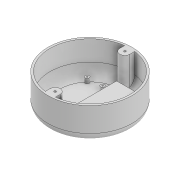
# Autodesk Inventor part: OrTak
Saved by Autodesk Inventor 2022 (Build 260153000, 153)
## iProperties
Created: 2023-02-07
Part Number: OrTak
Material: Generic
Document SubType Name: Modeling
Designer: MVeszpremi
Density: 1 g/cm^3
Appearance: Default
Author: MVeszpremi
Autodesk Inventor part; units mm, degrees
ref_plane "YZ Plane" through (0, 0, 0) normal (1, 0, 0) x (0, 1, 0)
ref_plane "XZ Plane" through (0, 0, 0) normal (0, 1, 0) x (-1, 0, 0)
ref_plane "XY Plane" through (0, 0, 0) normal (0, 0, 1) x (1, 0, 0)
sketch "Sketch1" plane through (0, 0, 0) normal (0, 1, 0) x (-1, 0, 0)
  circle A0 centre (0, 0) radius 62.5
  dimension "d0" = 125
  constraints: 1 centre point, 1 coincident
  measures "d0" diameter of A0
extrude "Extrusion1" add sketch "Sketch1" along normal blind 3
sketch "Sketch2" plane through (0, 3, 0) normal (0, 1, 0) x (1, 0, 0)
  line L0 (-33.1736, -29) -> (-10.1736, -29)
  line L1 (-10.1736, -29) -> (-10.1736, 29)
  line L2 (-10.1736, 29) -> (-33.1736, 29)
  line L3 (-33.1736, 29) -> (-33.1736, -29)
  line L4 (-33.1736, -29) -> (-10.1736, 29) construction
  line L5 (-10.1736, -29) -> (-33.1736, 29) construction
  circle A0 centre (-33.1736, -29) radius 3
  circle A1 centre (-33.1736, 29) radius 3
  circle A2 centre (-10.1736, 29) radius 3
  circle A3 centre (-10.1736, -29) radius 3
  circle A4 centre (-33.1736, -29) radius 0.95
  circle A5 centre (-33.1736, 29) radius 0.95
  circle A6 centre (-10.1736, 29) radius 0.95
  circle A7 centre (-10.1736, -29) radius 0.95
  point P0 (0, 0)
  point P1 (-21.6736, 0)
  dimension "d4" = 58
  dimension "d5" = 23
  dimension "d6" = 6
  dimension "d7" = 6
  dimension "d8" = 6
  dimension "d9" = 6
  dimension "d10" = 1.9
  dimension "d11" = 1.9
  dimension "d12" = 1.9
  dimension "d13" = 1.9
  constraints: 12 end point, 8 centre point, 8 coincident, 2 midpoint, 2 parallel, 1 horizontal, 1 perpendicular
  measures "d4" distance of L2.end L0.start
  measures "d5" distance of L1.end L2.end
  measures "d6" diameter of A0
  measures "d7" diameter of A1
  measures "d8" diameter of A2
  measures "d9" diameter of A3
  measures "d10" diameter of A4
  measures "d11" diameter of A7
  measures "d12" diameter of A6
  measures "d13" diameter of A5
extrude "Extrusion2" add sketch "Sketch2" along normal blind 7 contours A4 L3 A0 L0 | L0 A0 L3 A4 | A3 L1 A7 L0 | L0 A7 L1 A3 | A1 L2 A5 L3 | L3 A5 L2 A1 | A2 L2 A6 L1 | L1 A6 L2 A2
sketch "Sketch3" plane through (0, 3, 0) normal (0, 1, 0) x (1, 0, 0)
  line L0 (12.1501, -27.5) -> (39.6501, -27.5)
  line L1 (39.6501, -27.5) -> (39.6501, 27.5)
  line L2 (39.6501, 27.5) -> (12.1501, 27.5)
  line L3 (12.1501, 27.5) -> (12.1501, -27.5)
  line L4 (12.1501, -27.5) -> (39.6501, 27.5) construction
  line L5 (39.6501, -27.5) -> (12.1501, 27.5) construction
  line L6 (42.6501, -30.5) -> (9.1501, -30.5)
  line L7 (9.1501, -30.5) -> (9.1501, 30.5)
  line L8 (9.1501, 30.5) -> (42.6501, 30.5)
  line L9 (42.6501, 30.5) -> (42.6501, -30.5)
  line L10 (42.6501, -30.5) -> (9.1501, 30.5) construction
  line L11 (9.1501, -30.5) -> (42.6501, 30.5) construction
  circle A0 centre (25.9001, -27.5) radius 10.75
  circle A1 centre (25.9001, -27.5) radius 13.75
  point P0 (0, 0)
  point P1 (25.9001, 0)
  point P2 (15.1501, -27.5)
  point P3 (36.6501, -27.5)
  point P4 (12.4813, -30.5)
  point P5 (39.3188, -30.5)
  dimension "d16" = 55
  dimension "d17" = 27.5
  dimension "d18" = 3
  dimension "d19" = 3
  dimension "d20" = 3
  constraints: 24 end point, 5 midpoint, 4 parallel, 2 horizontal, 2 perpendicular, 1 centre point, 1 coincident, 3 other
  measures "d16" distance of L2.end L0.start
  measures "d17" distance of L1.end L2.end
  measures "d18" distance between parallel lines of L3 L7
  measures "d19" distance between parallel lines of L8 L2
extrude "Extrusion3" cut sketch "Sketch3" against normal blind 7 contours A0 L0 A1 | A0 L6 L0 | L0 A0 | A1 L3 L2 L1 | A0 L6
extrude "Extrusion4" add sketch "Sketch3" along normal blind 19 contours L0 A1 L6 A0 | L1 L2 L3 A1 L6 L7 L8 L9 | A0 L6 A1 L0 | L6 A1 A0
sketch "Sketch4" plane through (0, 22, 0) normal (0, 1, 0) x (1, 0, 0)
  line L0 (39.3188, -30.5) -> (42.6501, -30.5) projected
  line L1 (42.6501, -30.5) -> (42.6501, 30.5) projected
  line L2 (42.6501, 30.5) -> (9.1501, 30.5) projected
  line L3 (9.1501, 30.5) -> (9.1501, -30.5) projected
  line L4 (9.1501, -30.5) -> (12.4813, -30.5) projected
  arc A0 (12.4813, -30.5) -> (39.3188, -30.5) centre (25.9001, -27.5) ccw projected
  arc A1 (15.1501, -27.5) -> (36.6501, -27.5) centre (25.9001, -27.5) ccw projected
  line L5 (15.1501, -27.5) -> (12.1501, -27.5) projected
  line L6 (12.1501, -27.5) -> (12.1501, 27.5) projected
  line L7 (12.1501, 27.5) -> (39.6501, 27.5) projected
  line L8 (39.6501, 27.5) -> (39.6501, -27.5) projected
  line L9 (39.6501, -27.5) -> (36.6501, -27.5) projected
  point P0 (0, 0)
extrude "Extrusion5" add sketch "Sketch4" along normal blind 3 contours A0 L4 L3 L2 L1 L0 | L5 L6 L7 L8 L9 A1
sketch "Sketch5" plane through (0, 25, 0) normal (0, 1, 0) x (1, 0, 0)
  line L0 (12.1501, -27.5) -> (15.1501, -27.5) projected
  circle A0 centre (15.1501, -27.5) radius 2.5
  point P0 (0, 0)
  dimension "d27" = 5
  constraints: 1 centre point
  measures "d27" diameter of A0
extrude "Extrusion6" cut sketch "Sketch5" against normal blind 3
sketch "Sketch6" plane through (0, 3, 0) normal (0, 1, 0) x (1, 0, 0)
  circle A0 centre (0, 0) radius 62.5
  circle A1 centre (0, 0) radius 59.5
  circle A2 centre (0, 0) radius 62.5 projected
  dimension "d30" = 3
  constraints: 2 centre point, 2 coincident, 1 concentric
  measures "d30" radial gap between concentric circles of A0 A1
extrude "Extrusion7" add sketch "Sketch6" along normal blind 45
sketch "Sketch9" plane through (0, 48, 0) normal (0, 1, 0) x (1, 0, 0)
  circle A0 centre (0, -52) radius 7.5
  circle A1 centre (0, 0) radius 59.5 projected
  circle A2 centre (0, 52) radius 7.5
  circle A3 centre (0, -52) radius 1.45
  circle A4 centre (0, 52) radius 1.45
  line L0 (-7.5, -42.939) -> (7.5, -42.939)
  line L1 (7.5, -42.939) -> (7.5, -61.061)
  line L2 (7.5, -61.061) -> (-7.5, -61.061)
  line L3 (-7.5, -61.061) -> (-7.5, -42.939)
  line L4 (-7.5, -42.939) -> (7.5, -61.061) construction
  line L5 (7.5, -42.939) -> (-7.5, -61.061) construction
  line L6 (-7.5, 43.1519) -> (7.5, 43.1519)
  line L7 (7.5, 43.1519) -> (7.5, 60.8481)
  line L8 (7.5, 60.8481) -> (-7.5, 60.8481)
  line L9 (-7.5, 60.8481) -> (-7.5, 43.1519)
  line L10 (-7.5, 43.1519) -> (7.5, 60.8481) construction
  line L11 (7.5, 43.1519) -> (-7.5, 60.8481) construction
  point P0 (-7.5, 52)
  point P1 (7.5, 52)
  point P2 (7.5, 59.0254)
  point P3 (-7.5, 59.0254)
  point P4 (7.5, -52)
  point P5 (-7.5, -52)
  point P6 (-7.5, -59.0254)
  point P7 (7.5, -59.0254)
  dimension "d41" = 15
  dimension "d42" = 15
  dimension "d43" = 2.9
  dimension "d44" = 2.9
  constraints: 24 end point, 4 centre point, 4 midpoint, 4 parallel, 2 coincident, 2 horizontal, 2 perpendicular, 2 tangent, 1 point on line
  measures "d41" diameter of A0
  measures "d42" diameter of A2
  measures "d43" diameter of A3
  measures "d44" diameter of A4
extrude "Extrusion8" add sketch "Sketch9" against normal blind 45 contours A0 | L1 A1 A0 | A0 A1 L3 | A1 A2 L9 | L7 A2 A1 | A2
fillet "Fillet1" radius 15 3 edges at (-59.5, 3, 0) (44.6458, 3, -39.3319) (44.6458, 3, 39.3319)
fillet "Fillet2" radius 12 1 edges at (62.5, 0, 0)
sketch "Sketch10" plane through (0, 0, 0) normal (0, -1, 0) x (1, 0, 0)
  point P0 (0, 0)
sketch "Sketch12" plane through (0, 3, 0) normal (0, 1, 0) x (1, 0, 0)
  line L0 (9.1501, -30.5) -> (-0.8499, -30.5)
  line L1 (-0.8499, -30.5) -> (-0.8499, 30.5)
  line L2 (-0.8499, 30.5) -> (9.1501, 30.5)
  line L3 (9.1501, 30.5) -> (9.1501, -30.5)
  point P0 (0, 0)
  dimension "d52" = 10
  constraints: 8 end point, 2 parallel, 1 coincident, 1 horizontal, 1 perpendicular
  measures "d52" distance of L1.end L2.end
extrude "Extrusion10" add sketch "Sketch12" along normal blind 7.5
sketch "Sketch13" plane through (0, 0, 0) normal (0, -1, 0) x (1, 0, 0)
  circle A0 centre (9.6501, 0.0663) radius 5
  line L0 (9.6501, 5.0663) -> (22.1247, 5.0663)
  line L1 (22.1247, 5.0663) -> (22.1247, -4.9337)
  line L2 (22.1247, -4.9337) -> (9.6501, -4.9337)
  line L3 (9.6501, -4.9337) -> (9.6501, 5.0663)
  line L4 (12.1501, -27.5) -> (12.1501, 27.5) projected
  point P0 (0, 0)
  point P1 (12.1501, 5.0663)
  point P2 (12.1501, -4.9337)
  dimension "d55" = 10
  dimension "d56" = 2.5
  dimension "d57" = 2.5
  constraints: 8 end point, 2 parallel, 2 point on circle, 1 centre point, 1 horizontal, 1 perpendicular
  measures "d55" diameter of A0
  measures "d56" distance from line of L4 A0.centre
  measures "d57" distance between parallel lines of L4 L3
extrude "Extrusion11" cut sketch "Sketch13" against normal blind 5 contours L3 A0 | L0 L4 A0 | A0 L4 L3 | A0 L4 L2
sketch "Sketch14" plane through (0, 5, 0) normal (0, -1, 0) x (1, 0, 0)
  line L0 (9.1501, -30.5) -> (9.1501, 30.5) projected
  circle A0 centre (9.1501, 0) radius 1.45
  point P0 (0, 0)
  dimension "d60" = 2.9
  constraints: 1 centre point, 1 midpoint
  measures "d60" diameter of A0
extrude "Extrusion12" cut sketch "Sketch14" against normal blind 10
body "Solid1"
